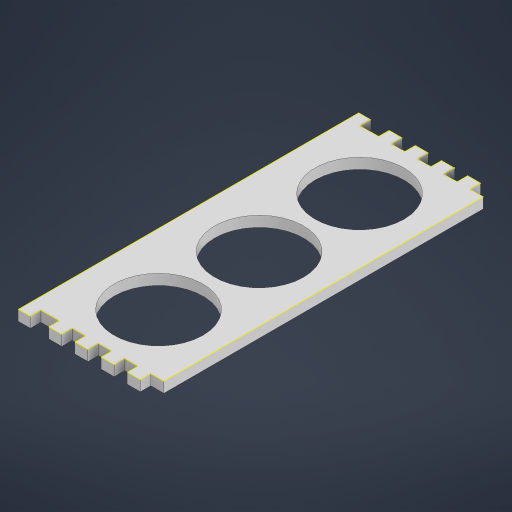
# Autodesk Inventor part: Angle Cover
Saved by Autodesk Inventor 2023 (Build 270158030, 158C)
## iProperties
Created: 2022-06-21
Part Number: Angle Cover
Material: Generic
Document SubType Name: Modeling
Designer: Simon
Density: 1 g/cm^3
Appearance: Default
Author: Simon
Autodesk Inventor part; units mm, degrees
ref_plane "YZ Plane" through (0, 0, 0) normal (1, 0, 0) x (0, 1, 0)
ref_plane "XZ Plane" through (0, 0, 0) normal (0, 1, 0) x (-1, 0, 0)
sketch "Sketch1" plane through (0, 0, 0) normal (0, 1, 0) x (-1, 0, 0)
  line L0 (-15, 0) -> (-15, 130)
  line L1 (-10, 0) -> (-10, 4)
  line L2 (-15, 4) -> (-10, 4)
  line L3 (-5, 0) -> (-10, 0)
  line L4 (-5, 0) -> (-5, 4)
  line L5 (-5, 4) -> (0, 4)
  line L6 (0, 0) -> (0, 4)
  line L7 (5, 0) -> (0, 0)
  line L8 (5, 0) -> (5, 4)
  line L9 (5, 4) -> (10, 4)
  line L10 (10, 0) -> (10, 4)
  line L11 (15, 0) -> (10, 0)
  line L12 (15, 0) -> (15, 4)
  line L13 (15, 4) -> (20, 4)
  line L14 (25, 0) -> (20, 0)
  line L15 (20, 0) -> (20, 4)
  line L16 (25, 0) -> (25, 4)
  line L17 (25, 4) -> (32, 4)
  line L18 (32, 0) -> (32, 4)
  line L19 (36.6188, 0) -> (32, 0)
  line L20 (36.6188, 0) -> (36.6188, 4)
  line L21 (36.6188, 4) -> (36.6188, 126)
  line L22 (36.6188, 126) -> (36.6188, 130)
  line L23 (32, 130) -> (36.6188, 130)
  line L24 (32, 126) -> (32, 130)
  line L25 (32, 126) -> (25, 126)
  line L26 (25, 126) -> (25, 130)
  line L27 (25, 130) -> (20, 130)
  line L28 (20, 126) -> (20, 130)
  line L29 (20, 126) -> (15, 126)
  line L30 (15, 126) -> (15, 130)
  line L31 (15, 130) -> (10, 130)
  line L32 (10, 126) -> (10, 130)
  line L33 (10, 126) -> (5, 126)
  line L34 (5, 126) -> (5, 130)
  line L35 (5, 130) -> (0, 130)
  line L36 (0, 126) -> (0, 130)
  line L37 (0, 126) -> (-5, 126)
  line L38 (-5, 126) -> (-5, 130)
  line L39 (-5, 130) -> (-10, 130)
  line L40 (-10, 126) -> (-10, 130)
  line L41 (-10, 126) -> (-15, 126)
  constraints: 84 end point
extrude "Extrusion1" add sketch "Sketch1" along normal blind 4
ref_plane "Work Plane1" through (15, 4, 130) normal (0.5, 0.866, 0) x (0, 0, -1)
sketch "Sketch5" plane through (0, 4, 0) normal (0, 1, 0) x (1, 0, 0)
  line L0 (10, 0) -> (5, 0) projected
  line L1 (5, 0) -> (5, -4) projected
  line L2 (5, -4) -> (0, -4) projected
  line L3 (0, -4) -> (0, 0) projected
  line L4 (0, 0) -> (-5, 0) projected
  line L5 (-5, 0) -> (-5, -4) projected
  line L6 (-5, -4) -> (-10, -4) projected
  line L7 (-10, -4) -> (-10, 0) projected
  line L8 (-10, 0) -> (-15, 0) projected
  line L9 (-15, 0) -> (-15, -4) projected
  line L10 (-15, -4) -> (-20, -4) projected
  line L11 (-20, -4) -> (-20, 0) projected
  line L12 (-20, 0) -> (-25, 0) projected
  line L13 (-25, 0) -> (-25, -4) projected
  line L14 (-25, -4) -> (-32, -4) projected
  line L15 (-32, -4) -> (-32, 0) projected
  line L16 (-32, 0) -> (-36.6188, 0) projected
  line L17 (-36.6188, 0) -> (-36.6188, -130) projected
  line L18 (-36.6188, -130) -> (-32, -130) projected
  line L19 (-32, -130) -> (-32, -126) projected
  line L20 (-32, -126) -> (-25, -126) projected
  line L21 (-25, -126) -> (-25, -130) projected
  line L22 (-25, -130) -> (-20, -130) projected
  line L23 (-20, -130) -> (-20, -126) projected
  line L24 (-20, -126) -> (-15, -126) projected
  line L25 (-15, -126) -> (-15, -130) projected
  line L26 (-15, -130) -> (-10, -130) projected
  line L27 (-10, -130) -> (-10, -126) projected
  line L28 (-10, -126) -> (-5, -126) projected
  line L29 (-5, -126) -> (-5, -130) projected
  line L30 (-5, -130) -> (0, -130) projected
  line L31 (0, -130) -> (0, -126) projected
  line L32 (0, -126) -> (5, -126) projected
  line L33 (5, -126) -> (5, -130) projected
  line L34 (5, -130) -> (10, -130) projected
  line L35 (10, -130) -> (10, -126) projected
  line L36 (10, -126) -> (15, -126) projected
  line L37 (15, -126) -> (15, -4) projected
  line L38 (15, -4) -> (10, -4) projected
  line L39 (10, -4) -> (10, 0) projected
sketch "Sketch6" plane through (0, 4, 0) normal (0, 1, 0) x (1, 0, 0)
  circle A0 centre (-9.6772, -26.5655) radius 17
  circle A1 centre (-9.6772, -64.9437) radius 17
  circle A2 centre (-9.6772, -103.3775) radius 17
  point P0 (0, 0)
  dimension "d16" = 34
  dimension "d17" = 34
  dimension "d18" = 34
  constraints: 3 centre point
  measures "d16" diameter of A0
  measures "d17" diameter of A1
  measures "d18" diameter of A2
extrude "Extrusion4" cut sketch "Sketch6" against normal blind 5.5
body "Solid1"
